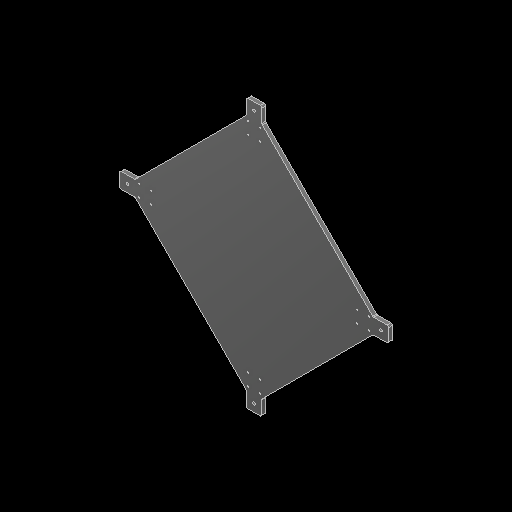
# Autodesk Inventor part: base_plate
Saved by Autodesk Inventor 2026.1 (Build 301233000, 233)
## iProperties
Created: 2025-09-14
Part Number: base_plate
Material: Aluminum 6061
Document SubType Name: Modeling
Designer: drago
Density: 2.7 g/cm^3
Appearance: Smooth - Black
Author: drago
Autodesk Inventor part; units mm, degrees
ref_plane "YZ Plane" through (0, 0, 0) normal (1, 0, 0) x (0, 1, 0)
ref_plane "XZ Plane" through (0, 0, 0) normal (0, 1, 0) x (-1, 0, 0)
ref_plane "XY Plane" through (0, 0, 0) normal (0, 0, 1) x (1, 0, 0)
sketch "Sketch2" plane through (0, 0, 0) normal (0, 0, 1) x (1, 0, 0)
  circle A0 centre (0, 0) radius 327.5 construction
  line L0 (-20, 307.5) -> (20, 307.5)
  line L1 (20, 307.5) -> (20, 347.5)
  line L2 (20, 347.5) -> (-20, 347.5)
  line L3 (-20, 347.5) -> (-20, 307.5)
  line L4 (-20, 307.5) -> (20, 347.5) construction
  line L5 (20, 307.5) -> (-20, 347.5) construction
  circle A1 centre (0, 327.5) radius 3.4
  circle A2 centre (-327.5, 0) radius 3.4
  line L6 (-347.5, 20) -> (-347.5, -20)
  line L7 (-347.5, -20) -> (-307.5, -20)
  line L8 (-307.5, -20) -> (-307.5, 20)
  line L9 (-307.5, 20) -> (-347.5, 20)
  line L10 (-307.5, 20) -> (-347.5, -20) construction
  line L11 (-307.5, -20) -> (-347.5, 20) construction
  circle A3 centre (0, -327.5) radius 3.4
  line L12 (-20, -347.5) -> (20, -347.5)
  line L13 (20, -347.5) -> (20, -307.5)
  line L14 (20, -307.5) -> (-20, -307.5)
  line L15 (-20, -307.5) -> (-20, -347.5)
  line L16 (-20, -307.5) -> (20, -347.5) construction
  line L17 (20, -307.5) -> (-20, -347.5) construction
  circle A4 centre (327.5, 0) radius 3.4
  line L18 (347.5, -20) -> (347.5, 20)
  line L19 (347.5, 20) -> (307.5, 20)
  line L20 (307.5, 20) -> (307.5, -20)
  line L21 (307.5, -20) -> (347.5, -20)
  line L22 (307.5, -20) -> (347.5, 20) construction
  line L23 (307.5, 20) -> (347.5, -20) construction
  line L24 (-20, 307.5) -> (-307.5, 20)
  line L25 (20, 307.5) -> (307.5, 20)
  line L26 (307.5, -20) -> (20, -307.5)
  line L27 (-20, -307.5) -> (-307.5, -20)
  line L28 (-307.5, 20) -> (307.5, 20)
  line L29 (-307.5, -20) -> (307.5, -20)
  line L30 (-20, 307.5) -> (-20, -307.5)
  line L31 (20, 307.5) -> (20, -307.5)
  line L32 (-299.2157, -28.2843) -> (28.2843, 299.2157)
  line L33 (-28.2843, 299.2157) -> (299.2157, -28.2843)
  line L34 (299.2157, 28.2843) -> (-28.2843, -299.2157)
  line L35 (-299.2157, 28.2843) -> (28.2843, -299.2157)
  line L36 (260.6, 21.1) -> (302.8, 21.1) construction
  line L37 (302.8, 21.1) -> (302.8, -21.1) construction
  line L38 (302.8, -21.1) -> (260.6, -21.1) construction
  line L39 (260.6, -21.1) -> (260.6, 21.1) construction
  line L40 (260.6, 21.1) -> (302.8, -21.1) construction
  line L41 (302.8, 21.1) -> (260.6, -21.1) construction
  circle A5 centre (297.2, 15.5) radius 1.6
  circle A6 centre (266.2, 15.5) radius 1.6
  circle A7 centre (266.2, -15.5) radius 1.6
  circle A8 centre (297.2, -15.5) radius 1.6
  circle A9 centre (-15.5, 266.2) radius 1.6
  circle A10 centre (-15.5, 297.2) radius 1.6
  circle A11 centre (15.5, 297.2) radius 1.6
  circle A12 centre (15.5, 266.2) radius 1.6
  circle A13 centre (-266.2, -15.5) radius 1.6
  circle A14 centre (-297.2, -15.5) radius 1.6
  circle A15 centre (-297.2, 15.5) radius 1.6
  circle A16 centre (-266.2, 15.5) radius 1.6
  circle A17 centre (15.5, -266.2) radius 1.6
  circle A18 centre (15.5, -297.2) radius 1.6
  circle A19 centre (-15.5, -297.2) radius 1.6
  circle A20 centre (-15.5, -266.2) radius 1.6
  point P0 (-250.9315, -20)
  point P1 (-20, -250.9315)
  point P2 (-20, -20)
  point P3 (20, -250.9315)
  point P4 (250.9315, -20)
  point P5 (20, -20)
  point P6 (250.9315, 20)
  point P7 (20, 250.9315)
  point P8 (20, 20)
  point P9 (-20, 250.9315)
  point P10 (-250.9315, 20)
  point P11 (-20, 20)
  point P12 (281.7, 0)
  dimension "d26" = 655
  dimension "d28" = 40
  dimension "d29" = 40
  dimension "d30" = 6.8
  dimension "d33" = 360
  dimension "d37" = 40
  dimension "d38" = 40
  dimension "d39" = 40
  dimension "d40" = 40
  dimension "d46" = 42.2
  dimension "d47" = 42.2
  dimension "d48" = 4.7
  dimension "d49" = 3.2
  dimension "d50" = 5.6
  dimension "d102" = 360
  dimension "d106" = 360
  constraints: 84 end point, 20 centre point, 9 perpendicular, 9 point on line, 5 parallel, 4 coincident, 4 midpoint, 2 horizontal, 1 collinear, 1 vertical alignment, 97 other
  measures "d28" distance of L2.end L1.end
  measures "d29" distance of L1.end L0.end
  measures "d30" diameter of A1
  measures "d37" distance between parallel lines of L32 L24
  measures "d38" distance between parallel lines of L33 L25
  measures "d39" distance between parallel lines of L26 L34
  measures "d40" distance between parallel lines of L27 L35
  measures "d46" distance of L36.start L36.end
  measures "d47" distance of L36.end L37.end
  measures "d48" distance between parallel lines of L20 L37
  measures "d49" diameter of A5
  measures "d50" distance from line of L36 A5.centre
extrude "Extrusion3" add sketch "Sketch2" against normal blind 10 contours L3 L2 L1 L0 | L30 L33 L24 | L0 L31 L32 L33 L30 | L25 L32 L31 | L33 L30 L32 L28 L35 L24 | L33 L32 L30 | L25 L34 L28 L33 L31 L32 | L31 L33 L32 | L35 L28 L24 | L32 L33 L31 L28 L30 | L30 L28 L32 | L25 L28 L34 | L33 L28 L31 | L28 L35 L32 L29 L8 | L8 L7 L6 L9 | L28 L32 L35 | L30 L29 L35 L32 L28 | L28 L31 L29 L30 | L19 L18 L21 L20 | L20 L29 L33 L34 L28 | L34 L33 L28 | L28 L33 L34 L29 L31 | L29 L32 L27 | L35 L29 L32 | L30 L35 L29 | L29 L31 L34 L35 L30 | L26 L33 L29 | L33 L29 L34 | L29 L34 L31 | L32 L29 L35 L30 L34 L27 | L35 L34 L30 | L26 L35 L31 L34 L29 L33 | L31 L35 L34 | L34 L30 L27 | L34 L35 L31 L14 L30 | L26 L31 L35 | L14 L13 L12 L15 | A5 | A6 | A7 | A8 | A9 | A10 | A11 | A12 | A13 | A14 | A15 | A16 | A17 | A18 | A19 | A20
fillet "Fillet5" radius 4 16 edges at (-307.5, 20, -5) (-347.5, 20, -5) (-347.5, -20, -5) (-20, -347.5, -5) (20, -347.5, -5) (-20, -307.5, -5) (-20, 347.5, -5) (307.5, -20, -5) (347.5, -20, -5) (347.5, 20, -5) (20, 307.5, -5) (20, 347.5, -5) (307.5, 20, -5) (-20, 307.5, -5) (-307.5, -20, -5) (20, -307.5, -5)
extrude "Extrusion6" cut sketch "Sketch2" against normal blind 10 contours A5 | A6 | A7 | A8 | A9 | A10 | A11 | A12 | A13 | A14 | A15 | A16 | A17 | A18 | A19 | A20
equation "\"d26\" = ring_outer_diam + bar_width"
equation "\"d28\" = bar_width"
equation "\"d29\" = bar_width"
equation "\"d30\" = bar_hole_diam"
equation "\"d37\" = bar_width"
equation "\"d38\" = bar_width"
equation "\"d39\" = bar_width"
equation "\"d40\" = bar_width"
equation "\"d46\" = motor_width"
equation "\"d47\" = motor_width"
equation "\"d48\" = dist_motor_bar"
equation "\"d35\" = base_plate_thick"
equation "\"ring_inner_diam\" = 565"
equation "\"bar_width\" = 40"
equation "\"bar_hole_diam\" = 6.8"
equation "\"ring_outer_diam\" = 615"
equation "\"base_plate_thick\" = 10"
equation "\"motor_width\" = 42.2"
equation "\"dist_motor_bar\" = 4.7"
equation "\"motor_hole_diam\" = 3.2"
equation "\"motor_hole_edge_dist\" = 5.6"
body "Solid2"
